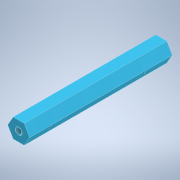
# Autodesk Inventor part: 6cmM3Standoff
Saved by Autodesk Inventor 2021 (Build 250183000, 183)
## iProperties
Created: 2020-03-11
Part Number: 6cmM3Standoff
Material: Generic
Document SubType Name: Modeling
Designer: elmar
Density: 1 g/cm^3
Appearance: Turquoise
Author: elmar
Autodesk Inventor part; units mm, degrees
ref_plane "YZ Plane" through (0, 0, 0) normal (1, 0, 0) x (0, 1, 0)
ref_plane "XZ Plane" through (0, 0, 0) normal (0, 1, 0) x (-1, 0, 0)
ref_plane "XY Plane" through (0, 0, 0) normal (0, 0, 1) x (1, 0, 0)
sketch "Sketch1" plane through (0, 0, 0) normal (0, 0, 1) x (1, 0, 0)
  line L0 (-2.3094, 4) -> (2.3094, 4)
  line L1 (2.3094, 4) -> (4.6188, 0)
  line L2 (4.6188, 0) -> (2.3094, -4)
  line L3 (2.3094, -4) -> (-2.3094, -4)
  line L4 (-2.3094, -4) -> (-4.6188, 0)
  line L5 (-4.6188, 0) -> (-2.3094, 4)
  point P0 (0, 0)
  point P1 (0, 0)
  dimension "d0" = 8
  constraints: 12 end point, 1 coincident, 1 horizontal, 13 other
  measures "d0" distance between parallel lines of L3 L0
extrude "Extrusion1" add sketch "Sketch1" along normal blind 60
sketch "Sketch2" plane through (0, 0, 0) normal (0, 0, -1) x (-1, 0, 0)
  point P0 (0, 0)
hole "Hole1" at (0, 0, 0) direction (0, 0, 1) diameter 3 end through all
sketch "Sketch5" plane through (0, 0, 0) normal (0, 1, 0) x (-1, 0, 0)
  line L0 (2.3094, 0) -> (2.3094, 60) projected
  line L1 (-2.3094, 0) -> (-2.3094, 60) projected
  line L2 (2.3094, 10) -> (-2.3094, 10)
  line L3 (-2.3094, 10) -> (-2.3094, 50)
  line L4 (-2.3094, 50) -> (2.3094, 50)
  line L5 (2.3094, 50) -> (2.3094, 10)
  point P0 (0, 0)
  point P1 (2.3094, 50)
  dimension "d30" = 10
  dimension "d31" = 40
  constraints: 8 end point, 2 parallel, 2 point on line, 1 horizontal, 1 perpendicular
  measures "d30" distance from line of L0.start L2
  measures "d31" distance between parallel lines of L4 L2
extrude "Extrusion2" add sketch "Sketch5" along normal mid plane 4
sketch "Sketch6" plane through (4.6188, 0, 60) normal (0.866, -0.5, 0) x (0, 0, -1)
  line L0 (72, -2.3094) -> (-12, -2.3094) projected
  line L1 (10, -1.1547) -> (10, -3.4641) projected
  line L2 (50, -0.8094) -> (50, -3.8094) projected
  point P0 (60, -2.3094)
  point P1 (10, -2.3094)
  point P2 (50, -2.3094)
  constraints: 2 midpoint, 1 point on line
thread "Thread2" size "M3x0.5" class "6H" standard "ANSI Metric M Profile" full length
thread "Thread3" size "M3x0.5" class "6H" standard "ANSI Metric M Profile" full length
sketch "Sketch8" plane through (0, 0, 50) normal (1, 0, 0) x (0, 1, 0)
  line L0 (1.5, 0) -> (1.5, 10)
  line L1 (1.5, 10) -> (1.1293, 10)
  line L2 (1.1293, 10) -> (1.1293, 0)
  line L3 (1.1293, 0) -> (1.5, 0)
  line L4 (0, -62) -> (0, 22) projected
  constraints: 8 end point
revolve "Revolution2" add sketch "Sketch8" angle 360 about axis through (0, 0, 50) along (0, 0, 1) separate body
sketch "Sketch7" plane through (0, 1.5, 50) normal (-1, 0, 0) x (0, 0, 1)
  line L0 (-0.2918, -0.0255) -> (-0.2501, -0.0255) construction
  line L1 (0.0416, -0.3456) -> (-0.0001, -0.4257) construction
  line L2 (-0.5001, -0.4257) -> (-0.5418, -0.3456) construction
  line L3 (-0.2084, -0.0255) -> (-0.2501, 0.0546) construction
  line L4 (-0.2501, 0.0546) -> (-0.2918, -0.0255) construction
  line L5 (-0.5001, -0.4257) -> (-0.4584, -0.3456) construction
  line L6 (-0.2084, -0.0255) -> (-0.0418, -0.3456)
  line L7 (-0.5418, -0.3456) -> (-0.4584, -0.3456) construction
  arc A0 (-0.5418, -0.3456) -> (-0.5001, -0.3709) centre (-0.5001, -0.3239) ccw construction
  line L8 (0.0416, -0.3456) -> (-0.0418, -0.3456) construction
  line L9 (-0.5001, -0.4257) -> (-0.5001, -0.3456) construction
  line L10 (-0.0001, -0.4257) -> (-0.0001, -0.3456) construction
  line L11 (-0.2501, 0.0546) -> (-0.2501, -0.0002) construction
  line L12 (-0.5001, -0.3709) -> (-0.0001, -0.3709)
  arc A1 (-0.5001, -0.3709) -> (-0.4584, -0.3456) centre (-0.5001, -0.3239) ccw
  line L13 (-0.0418, -0.3456) -> (-0.0001, -0.4257) construction
  line L14 (-0.4584, -0.3456) -> (-0.2918, -0.0255)
  line L15 (-0.0001, -0.0002) -> (-0.0001, 0.0177)
  line L16 (-0.0001, 0.0177) -> (-0.0001, -0.0002)
  line L17 (-0.0001, -0.0002) -> (0.0334, -0.0002)
  arc A2 (-0.0418, -0.3456) -> (-0.0001, -0.3709) centre (-0.0001, -0.3239) ccw
  arc A3 (-0.0001, -0.3709) -> (0.0416, -0.3456) centre (-0.0001, -0.3239) ccw construction
  arc A4 (-0.2501, -0.0002) -> (-0.2918, -0.0255) centre (-0.2501, -0.0471) ccw
  arc A5 (-0.2084, -0.0255) -> (-0.2501, -0.0002) centre (-0.2501, -0.0471) ccw
  line L18 (-0.2501, -0.0002) -> (-0.2501, -0.0255) construction
  line L19 (-0.2501, -0.0255) -> (-0.2084, -0.0255) construction
  dimension "d45" = 55
  dimension "d46" = 0.08
  dimension "d47" = 0.08
  dimension "Sketch7_ThreadOffset" = 0
  dimension "Sketch7_MajorRadius" = 0.3707
  dimension "d50" = 0.5
  dimension "Sketch7_MinorRadius" = 0
  constraints: 40 end point, 12 point on circle, 10 parallel, 8 tangent, 6 centre point, 6 collinear, 2 midpoint, 2 point on line, 1 horizontal, 1 perpendicular, 3 other
  measures "d45" angle of L6 L14
  measures "d46" distance of L3.end L0.end
  measures "d47" distance of L1.end L10.end
  measures "Sketch7_ThreadOffset" distance between parallel lines of L15 L10
  measures "Sketch7_MajorRadius" distance from line of L12 L15.start
  measures "d50" distance from line of L1.end L9
  measures "Sketch7_MinorRadius" distance edge to line of A5 L17
coil "Coil2" sketch "Sketch7" operation cut axis through (0, 0, 50) along (0, 0, 1) pitch 0.5005 turns 21.978022 hand right bodies 2
sketch "Sketch10" plane through (0, 0, 0) normal (1, 0, 0) x (0, 1, 0)
  line L0 (1.5, 0) -> (1.5, 10)
  line L1 (1.5, 10) -> (1.1293, 10)
  line L2 (1.1293, 10) -> (1.1293, 0)
  line L3 (1.1293, 0) -> (1.5, 0)
  line L4 (0, -12.6877) -> (0, 72.3091) projected
  constraints: 8 end point
revolve "Revolution3" add sketch "Sketch10" angle 360 about axis through (0, 0, 0) along (0, 0, 1) separate body
sketch "Sketch9" plane through (0, 1.5, 0) normal (-1, 0, 0) x (0, 0, 1)
  line L0 (-0.2918, -0.0255) -> (-0.2501, -0.0255) construction
  line L1 (0.0416, -0.3456) -> (-0.0001, -0.4257) construction
  line L2 (-0.5001, -0.4257) -> (-0.5418, -0.3456) construction
  line L3 (-0.2084, -0.0255) -> (-0.2501, 0.0546) construction
  line L4 (-0.2501, 0.0546) -> (-0.2918, -0.0255) construction
  line L5 (-0.5001, -0.4257) -> (-0.4584, -0.3456) construction
  line L6 (-0.2084, -0.0255) -> (-0.0418, -0.3456)
  line L7 (-0.5418, -0.3456) -> (-0.4584, -0.3456) construction
  arc A0 (-0.5418, -0.3456) -> (-0.5001, -0.3709) centre (-0.5001, -0.3239) ccw construction
  line L8 (0.0416, -0.3456) -> (-0.0418, -0.3456) construction
  line L9 (-0.5001, -0.4257) -> (-0.5001, -0.3456) construction
  line L10 (-0.0001, -0.4257) -> (-0.0001, -0.3456) construction
  line L11 (-0.2501, 0.0546) -> (-0.2501, -0.0002) construction
  line L12 (-0.5001, -0.3709) -> (-0.0001, -0.3709)
  arc A1 (-0.5001, -0.3709) -> (-0.4584, -0.3456) centre (-0.5001, -0.3239) ccw
  line L13 (-0.0418, -0.3456) -> (-0.0001, -0.4257) construction
  line L14 (-0.4584, -0.3456) -> (-0.2918, -0.0255)
  line L15 (-0.0001, -0.0002) -> (-0.0001, 0.0177)
  line L16 (-0.0001, 0.0177) -> (-0.0001, -0.0002)
  line L17 (-0.0001, -0.0002) -> (0.0334, -0.0002)
  arc A2 (-0.0418, -0.3456) -> (-0.0001, -0.3709) centre (-0.0001, -0.3239) ccw
  arc A3 (-0.0001, -0.3709) -> (0.0416, -0.3456) centre (-0.0001, -0.3239) ccw construction
  arc A4 (-0.2501, -0.0002) -> (-0.2918, -0.0255) centre (-0.2501, -0.0471) ccw
  arc A5 (-0.2084, -0.0255) -> (-0.2501, -0.0002) centre (-0.2501, -0.0471) ccw
  line L18 (-0.2501, -0.0002) -> (-0.2501, -0.0255) construction
  line L19 (-0.2501, -0.0255) -> (-0.2084, -0.0255) construction
  dimension "d63" = 55
  dimension "d64" = 0.08
  dimension "d65" = 0.08
  dimension "Sketch9_ThreadOffset" = 0
  dimension "Sketch9_MajorRadius" = 0.3707
  dimension "d68" = 0.5
  dimension "Sketch9_MinorRadius" = 0
  constraints: 40 end point, 12 point on circle, 10 parallel, 8 tangent, 6 centre point, 6 collinear, 2 midpoint, 2 point on line, 1 horizontal, 1 perpendicular, 3 other
  measures "d63" angle of L6 L14
  measures "d64" distance of L3.end L0.end
  measures "d65" distance of L1.end L10.end
  measures "Sketch9_ThreadOffset" distance between parallel lines of L15 L10
  measures "Sketch9_MajorRadius" distance from line of L12 L15.start
  measures "d68" distance from line of L1.end L9
  measures "Sketch9_MinorRadius" distance edge to line of A5 L17
coil "Coil3" sketch "Sketch9" operation cut axis through (0, 0, 0) along (0, 0, 1) pitch 0.5005 turns 21.978022 hand right bodies 3
hole "Hole3" at (3.4641, -2, 50) at (3.4641, -2, 10) direction (-0.866, 0.5, 0) diameter 1 end through all bodies 1 2 3
equation "\"d45\" = d52"
equation "\"d46\" = 0.160083 * Sketch7_Pitch"
equation "\"d47\" = 0.160083 * Sketch7_Pitch"
equation "\"d50\" = Sketch7_Pitch"
equation "\"d63\" = d70"
equation "\"d64\" = 0.160083 * Sketch9_Pitch"
equation "\"d65\" = 0.160083 * Sketch9_Pitch"
equation "\"d68\" = Sketch9_Pitch"
equation "\"d19\" = 55deg"
equation "\"Sketch3_Pitch\" = 0.5"
equation "\"d52\" = 55deg"
equation "\"Sketch7_Pitch\" = 0.5"
equation "\"d70\" = 55deg"
equation "\"Sketch9_Pitch\" = 0.5"
body "Solid1"
body "Solid3"
body "Solid4"
